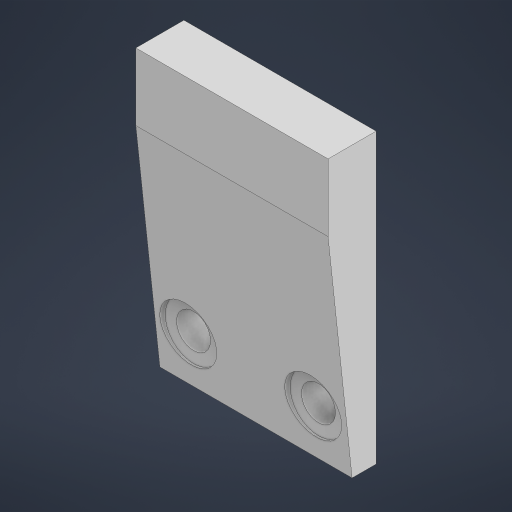
# Autodesk Inventor part: Drone_Launcher_Stopper
Saved by Autodesk Inventor 2023 (Build 270158000, 158)
## iProperties
Created: 2024-02-18
Part Number: Drone_Launcher_Stopper
Material: Generic
Document SubType Name: Modeling
Designer: kelle
Density: 1 g/cm^3
Appearance: Default
Author: kelle
Autodesk Inventor part; units mm, degrees
ref_plane "YZ Plane" through (0, 0, 0) normal (1, 0, 0) x (0, 1, 0)
ref_plane "XZ Plane" through (0, 0, 0) normal (0, 1, 0) x (-1, 0, 0)
sketch "Sketch1" plane through (0, 0, 0) normal (0, 0, 1) x (1, 0, 0)
  line L0 (12.7, -19.05) -> (-12.7, -19.05)
  line L1 (-12.7, -19.05) -> (-12.7, 19.05)
  line L2 (-12.7, 19.05) -> (12.7, 19.05)
  line L3 (12.7, 19.05) -> (12.7, -19.05)
  line L4 (12.7, -19.05) -> (-12.7, 19.05) construction
  line L5 (-12.7, -19.05) -> (12.7, 19.05) construction
  circle A0 centre (-8.255, -12.7) radius 2.25
  circle A1 centre (8.255, -12.7) radius 2.25
  line L6 (0, 19.05) -> (0, -19.05) construction
  line L7 (-6.005, 19.05) -> (-6.005, -19.05) construction
  line L8 (6.005, 19.05) -> (6.005, -19.05) construction
  line L9 (-6.005, 19.05) -> (2.4874, 19.05) construction
  circle A2 centre (-8.255, -12.7) radius 3.75
  circle A3 centre (8.255, -12.7) radius 3.75
  point P0 (0, 0)
  point P1 (0, 13.045)
  dimension "d0" = 25.4
  dimension "d1" = 38.1
  dimension "d2" = 4.5
  dimension "d3" = 4.5
  dimension "d4" = 8.255
  dimension "d5" = 8.255
  dimension "d6" = 6.35
  dimension "d7" = 6.35
  dimension "d14" = 7.5
  dimension "d15" = 7.5
  constraints: 20 end point, 5 point on line, 4 centre point, 4 midpoint, 3 perpendicular, 2 coincident, 2 horizontal, 2 parallel
  measures "d0" distance of L1.end L2.end
  measures "d1" distance of L0.end L1.end
  measures "d2" diameter of A0
  measures "d3" diameter of A1
  measures "d4" distance from line of L6 A0.centre
  measures "d5" distance from line of L6 A1.centre
  measures "d6" distance from line of L0 A1.centre
  measures "d7" distance from line of L0 A0.centre
  measures "d14" diameter of A2
  measures "d15" diameter of A3
extrude "Extrusion1" add sketch "Sketch1" along normal blind 6.35 contours L0 L1 L2 L3 | A2 | A3
sketch "Sketch2" plane through (12.7, -19.05, 0) normal (1, 0, 0) x (0, 0, -1)
  line L0 (-6.35, 32.095) -> (-6.35, 38.1) projected
  line L1 (0, 38.1) -> (0, 0) projected
  line L2 (-6.35, 38.1) -> (0, 38.1)
  line L3 (0, 38.1) -> (0, 29.21)
  line L4 (0, 29.21) -> (-6.35, 29.21)
  line L5 (-6.35, 29.21) -> (-6.35, 38.1)
  line L6 (-6.35, 29.21) -> (-3.175, 0)
  line L7 (0, 0) -> (-6.35, 0) projected
  line L8 (-3.175, 0) -> (0, 0)
  line L9 (-6.35, 4.1) -> (0, 4.1) projected
  line L10 (0, 0) -> (0, 38.1) projected
  line L11 (0, 38.1) -> (-6.35, 38.1) projected
  line L12 (-6.35, 0) -> (-6.35, 38.1) projected
  line L13 (0, 0) -> (-6.35, 0) projected
  point P0 (0, 19.05)
  dimension "d11" = 8.89
  constraints: 12 end point, 2 horizontal, 2 parallel, 1 perpendicular, 1 point on line
  measures "d11" distance of L2.end L3.end
extrude "Extrusion2" cut sketch "Sketch2" against normal through all contours L6 L9 L12 | L6 L7 L12 L9
ref_plane "Work Plane1" through (12.7, 14.605, 6.35) normal (0, 0, 1) x (1, 0, 0)
sketch "Sketch3" plane through (12.7, 14.605, 6.35) normal (0, 0, 1) x (1, 0, 0)
  line L0 (-25.4, -33.655) -> (-25.4, -4.445) projected
  line L1 (0, -33.655) -> (-25.4, -33.655) projected
  line L2 (0, -4.445) -> (0, -33.655) projected
  line L3 (-25.4, -4.445) -> (0, -4.445) projected
  circle A0 centre (-4.445, -27.305) radius 2.25 projected
  circle A1 centre (-20.955, -27.305) radius 2.25 projected
  circle A2 centre (-20.955, -27.305) radius 2.25 projected
  circle A3 centre (-20.955, -27.305) radius 3.75
  circle A4 centre (-4.445, -27.305) radius 3.75
  point P0 (-12.7, -14.605)
  dimension "d16" = 7.5
  dimension "d17" = 7.5
  constraints: 2 centre point, 2 coincident
  measures "d16" diameter of A3
  measures "d17" diameter of A4
extrude "Extrusion3" cut sketch "Sketch3" against normal blind 3.175 contours A1 | A3 | A4
body "Solid1"
